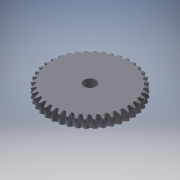
# Autodesk Inventor part: Worm Gear
Saved by Autodesk Inventor 2016 (Build 200138000, 138)
## iProperties
Created: 2015-06-13
Part Number: Worm Gear
Material: Steel, Mild
Document SubType Name: Modeling
Designer: steele
Categories: <?xml version="1.0" encoding="UTF-16"?> <MemberInstance><Categories><FamilyTemplate><FamilyTemplateParameter ValueType="xs:double" Id="1" ObjectReferenceKey="da_z" ObjectType="kUserParameterObject"/><FamilyTemplateParameter ValueType="xs:double" Id="2" ObjectReferenceKey="da_b" ObjectType="kUserParameterObject"/><FamilyTemplateParameter ValueType="xs:double" Id="3" ObjectReferenceKey="da_beta" ObjectType="kUserParameterObject"/><FamilyTemplateParameter ValueType="xs:double" Id="4" ObjectReferenceKey="da_m" ObjectType="kUserParameterObject"/><FamilyTemplateParameter ValueType="xs:double" Id="5" ObjectReferenceKey="da_alpha" ObjectType="kUserParameterObject"/><FamilyTemplateParameter ValueType="xs:double" Id="6" ObjectReferenceKey="da_da" ObjectType="kUserParameterObject"/><FamilyTemplateParameter ValueType="xs:double" Id="7" ObjectReferenceKey="da_aw" ObjectType="kUserParameterObject"/><FamilyTemplateParameter ValueType="xs:double" Id="8" ObjectReferenceKey="da_px" ObjectType="kUserParameterObject"/><FamilyTemplateParameter ValueType="xs:double" Id="9" ObjectReferenceKey="da_d" ObjectType="kUserParameterObject"/><FamilyTemplateParameter ValueType="xs:double" Id="10" ObjectReferenceKey="da_dae" ObjectType="kUserParameterObject"/><FamilyTemplateParameter ValueType="xs:double" Id="11" ObjectReferenceKey="da_fi" ObjectType="kUserParameterObject"/><FamilyTemplateParameter ValueType="xs:string" Id="12" ObjectReferenceKey="EAIAABAAAAAWFwAAAAAAAIAAAAAAAAAA" ObjectType="83910656" SubObjectId="SurfaceGeometry"/></FamilyTemplate><ParamToTemplateMap><ParamToTemplate CategoryParameter="//CategoryParameter[@InternalName='046C89C9-8512-4d59-83FE-43B91F4F132A']" TemplateParameter="1"/><ParamToTemplate CategoryParameter="//CategoryParameter[@InternalName='2552DF32-E462-4b46-AEBF-C6C7768E72AC']" TemplateParameter="2"/><ParamToTemplate CategoryParameter="//CategoryParameter[@InternalName='C9EE641D-15FC-4fae-A226-E94C4372FDD7']" TemplateParameter="3"/><ParamToTemplate><ParamToTemplate CategoryParameter="//CategoryParameter[@InternalName='00B6519A-459B-49c7-AD84-2E56D39A5744']" ConstantValue="0.000000"/></ParamToTemplate><ParamToTemplate><ParamToTemplate CategoryParameter="//CategoryParameter[@InternalName='04B31F0E-C7A6-4894-AA32-9629BEFACF47']" ConstantValue="1.000000"/></ParamToTemplate><ParamToTemplate><ParamToTemplate CategoryParameter="//CategoryParameter[@InternalName='43CBEC2E-7847-49e7-A936-2F7889FCB2D9']" ConstantValue="0.200000"/></ParamToTemplate><ParamToTemplate><ParamToTemplate CategoryParameter="//CategoryParameter[@InternalName='B1EFC894-105D-4ebd-86BF-FA20ED196853']" ConstantValue="0.266800"/></ParamToTemplate><ParamToTemplate><ParamToTemplate CategoryParameter="//CategoryParameter[@InternalName='51175063-3D10-4879-93E8-6246FE8B403D']" ConstantValue="2061532430.657340"/></ParamToTemplate><ParamToTemplate><ParamToTemplate CategoryParameter="//CategoryParameter[@InternalName='A3A52E27-4454-46a9-B0BD-C932399B70AF']" ConstantValue="0.300000"/></ParamToTemplate><ParamToTemplate CategoryParameter="//CategoryParameter[@InternalName='91B76062-C214-41d9-B1B9-14D2AB99603D']" TemplateParameter="4"/><ParamToTemplate CategoryParameter="//CategoryParameter[@InternalName='2D373A89-B862-43d6-8D0B-0CBF12AB9F6C']" TemplateParameter="5"/><ParamToTemplate CategoryParameter="//CategoryParameter[@InternalName='37777632-D6A2-4fac-9D53-DB8ACD95C989']" TemplateParameter="6"/><ParamToTemplate CategoryParameter="//CategoryParameter[@InternalName='FD1017F1-B727-4f7e-9707-0F86F1FF9423']" TemplateParameter="7"/><ParamToTemplate CategoryParameter="//CategoryParameter[@InternalName='3BF567DA-17EF-48d8-80EA-D119B07F6463']" TemplateParameter="8"/><ParamToTemplate CategoryParameter="//CategoryParameter[@InternalName='BF5A1E7E-5373-4a22-AAD3-F583781FCF3C']" TemplateParameter="9"/><ParamToTemplate CategoryParameter="//CategoryParameter[@InternalName='2A200944-5A8C-41ca-B96E-8520D2E510F1']" TemplateParameter="10"/><ParamToTemplate CategoryParameter="//CategoryParameter[@InternalName='E77AC4FD-7B43-4566-B0ED-7CA70B976BC8']" TemplateParameter="11"/><ParamToTemplate><ParamToTemplate CategoryParameter="//CategoryParameter[@InternalName='D4F72237-D604-435a-AD0B-F738B7463A00']" ConstantValue="110.000000"/></ParamToTemplate><ParamToTemplate><ParamToTemplate CategoryParameter="//CategoryParameter[@InternalName='9E1B4470-B2D3-4ff1-B813-535BB4CDF51A']" ConstantValue="1999479.615019"/></ParamToTemplate><ParamToTemplate><ParamToTemplate CategoryParameter="//CategoryParameter[@InternalName='A7A89E9A-52E6-4d4f-86CF-A81914F22AA4']" ConstantValue="250000000.000000"/></ParamToTemplate><ParamToTemplate><ParamToTemplate CategoryParameter="//CategoryParameter[@InternalName='B02FABAC-469F-4ad8-A219-DB4578299DF6']" ConstantValue="250000000.000000"/></ParamToTemplate><ParamToTemplate><ParamToTemplate CategoryParameter="//CategoryParameter[@InternalName='E6981962-40D5-4343-A0AD-C263FCC47E10']" ConstantValue="9.000000"/></ParamToTemplate><ParamToTemplate><ParamToTemplate CategoryParameter="//CategoryParameter[@InternalName='B958E99F-2BCD-4955-8634-793EB7B37B89']" ConstantValue="8.000000"/></ParamToTemplate><ParamToTemplate><ParamToTemplate CategoryParameter="//CategoryParameter[@InternalName='4AD49A87-569D-440f-A541-E3B52A6A9DCE']" ConstantValue="1219.200000"/></ParamToTemplate><ParamToTemplate><ParamToTemplate CategoryParameter="//CategoryParameter[@InternalName='4E5813A0-330D-4b41-BE23-D880B01A1D55']" ConstantValue="1654741.750360"/></ParamToTemplate><ParamToTemplate><ParamToTemplate CategoryParameter="//CategoryParameter[@InternalName='19EB8C86-AA88-4253-B4AA-2F5DF1CE171A']" ConstantValue="5515.805835"/></ParamToTemplate><ParamToTemplate CategoryParameter="//CategoryParameter[@InternalName='27C3BAF2-7550-4e4b-AE2C-0DB134B7D9B7']" TemplateParameter="12"/></ParamToTemplateMap><Category DisplayName="Gear" InternalName="DC85795E-93AB-48d5-8EEE-5A27447B64BD" Mnemonic="Gear"><CategoryParameter DisplayName="z" InternalName="046C89C9-8512-4d59-83FE-43B91F4F132A" Mnemonic="z"/><CategoryParameter DisplayName="b|.2|" InternalName="2552DF32-E462-4b46-AEBF-C6C7768E72AC" Mnemonic="b"/><CategoryParameter DisplayName="||b|" InternalName="C9EE641D-15FC-4fae-A226-E94C4372FDD7" Mnemonic="beta"/><CategoryParameter DisplayName="x" InternalName="00B6519A-459B-49c7-AD84-2E56D39A5744" Mnemonic="x"/><CategoryParameter DisplayName="a*" InternalName="04B31F0E-C7A6-4894-AA32-9629BEFACF47" Mnemonic="a"/><CategoryParameter DisplayName="c*" InternalName="43CBEC2E-7847-49e7-A936-2F7889FCB2D9" Mnemonic="c"/><CategoryParameter DisplayName="r|.f|*" InternalName="B1EFC894-105D-4ebd-86BF-FA20ED196853" Mnemonic="rf"/><CategoryParameter DisplayName="E" InternalName="51175063-3D10-4879-93E8-6246FE8B403D" Mnemonic="E"/><CategoryParameter DisplayName="||m|" InternalName="A3A52E27-4454-46a9-B0BD-C932399B70AF" Mnemonic="mi"/><Category DisplayName="WormGear" InternalName="1B25C7EF-093B-4025-B3D3-619CD2A4550C" Mnemonic="WormGear"><CategoryParameter DisplayName="m" InternalName="91B76062-C214-41d9-B1B9-14D2AB99603D" Mnemonic="m"/><CategoryParameter DisplayName="||a|" InternalName="2D373A89-B862-43d6-8D0B-0CBF12AB9F6C" Mnemonic="alpha"/><CategoryParameter DisplayName="d|.a|" InternalName="37777632-D6A2-4fac-9D53-DB8ACD95C989" Mnemonic="da"/><CategoryParameter DisplayName="a|.w|" InternalName="FD1017F1-B727-4f7e-9707-0F86F1FF9423" Mnemonic="aw"/><CategoryParameter DisplayName="p|.x|" InternalName="3BF567DA-17EF-48d8-80EA-D119B07F6463" Mnemonic="px"/><CategoryParameter DisplayName="d" InternalName="BF5A1E7E-5373-4a22-AAD3-F583781FCF3C" Mnemonic="d"/><CategoryParameter DisplayName="dae" InternalName="2A200944-5A8C-41ca-B96E-8520D2E510F1" Mnemonic="dae"/><CategoryParameter DisplayName="||d|" InternalName="E77AC4FD-7B43-4566-B0ED-7CA70B976BC8" Mnemonic="fi"/><CategoryParameter DisplayName="VHV" InternalName="D4F72237-D604-435a-AD0B-F738B7463A00" Mnemonic="VHV"/><CategoryParameter DisplayName="||s||.Hlim|" InternalName="9E1B4470-B2D3-4ff1-B813-535BB4CDF51A" Mnemonic="sHlim"/><CategoryParameter DisplayName="N|.Flim|" InternalName="A7A89E9A-52E6-4d4f-86CF-A81914F22AA4" Mnemonic="NFlim"/><CategoryParameter DisplayName="N|.Hlim|" InternalName="B02FABAC-469F-4ad8-A219-DB4578299DF6" Mnemonic="NHlim"/><CategoryParameter DisplayName="q|.F|" InternalName="E6981962-40D5-4343-A0AD-C263FCC47E10" Mnemonic="qF"/><CategoryParameter DisplayName="q|.H|" InternalName="B958E99F-2BCD-4955-8634-793EB7B37B89" Mnemonic="qH"/><CategoryParameter DisplayName="v|.max|" InternalName="4AD49A87-569D-440f-A541-E3B52A6A9DCE" Mnemonic="maxv"/><CategoryParameter DisplayName="S|.n|" InternalName="4E5813A0-330D-4b41-BE23-D880B01A1D55" Mnemonic="Sn"/><CategoryParameter DisplayName="K|.w|" InternalName="19EB8C86-AA88-4253-B4AA-2F5DF1CE171A" Mnemonic="Kw"/><CategoryParameter DisplayName="PitchDiameter" InternalName="27C3BAF2-7550-4e4b-AE2C-0DB134B7D9B7" Mnemonic="IDS_PITCHDIAM"/></Category></Category></Categories></MemberInstance>
Density: 7.86 g/cm^3
Appearance: Steel
CustomPartVersion: 1
Author: steele
Autodesk Inventor part; units mm, degrees
ref_plane "YZ Plane" through (0, 0, 0) normal (1, 0, 0) x (0, 1, 0)
ref_plane "XZ Plane" through (0, 0, 0) normal (0, 1, 0) x (-1, 0, 0)
ref_plane "XY Plane" through (0, 0, 0) normal (0, 0, 1) x (1, 0, 0)
ref_plane "Tooth Plane" through (0, -10, 0) normal (-0.0830455, 0, 0.9965458) x (0, 1, 0)
sketch "Base Body Sketch" plane through (0, 0, 0) normal (1, 0, 0) x (0, 1, 0)
  line L0 (0, -5.9267) -> (0, 5.9267) projected
  line L1 (0, 3.175) -> (20.8232, 3.175)
  line L2 (20.8232, 3.175) -> (22.7542, 2.2591)
  line L3 (-6.1383, 0) -> (36.83, 0) construction
  circle A0 centre (27.5167, 0) radius 5.2917
  line L4 (22.7542, 2.2591) -> (22.7542, -2.2591)
  line L5 (0, -3.175) -> (20.8232, -3.175)
  line L6 (0, 3.175) -> (0, -3.175)
  line L7 (20.8232, -3.175) -> (22.7542, -2.2591)
  dimension "d50" = 25.377
  dimension "d87" = 45.5083
  dimension "d89" = 10.5833
  dimension "d92" = 6.35
  dimension "d93" = 27.5167
  constraints: 14 end point, 3 symmetric about line, 2 perpendicular, 2 point on line, 1 centre point, 1 collinear
  measures "d50" angle of L2 L1
  measures "d87" diameter of L4 L0
  measures "d89" diameter of A0
  measures "d92" distance of L1.start L5.start
  measures "d93" distance from line of A0.centre L6
revolve "Base Body" add sketch "Base Body Sketch" angle 360 about axis through (0, 0, 0) along (0, 0, 1) picked at (22.6209, 0.3874) contours L0 L1 L2 A0 L7 L5 | A0 L2 L4 L7
revolve "Base Body2" cut sketch "Base Body Sketch" angle 360 about axis through (0, 0, 0) along (0, 0, 1) contours L7 L4 L2 A0 | A0 L2 L4 L7
sketch "Tooth Sketch" plane through (0, -10, 0) normal (-0.0830455, 0, 0.9965458) x (0, 1, 0)
  line L0 (10, 2.0436) -> (10, -2.0436) projected
  line L1 (-17.7707, 0) -> (-8.5843, 0) projected
  line L2 (-17.5167, 1.4597) -> (-17.5167, -1.4597)
  line L3 (-17.5167, -1.4597) -> (-12.4367, -1.4597)
  line L4 (-12.4367, -1.4597) -> (-9.8967, -0.5352)
  line L5 (-9.8967, -0.5352) -> (-9.8967, 0)
  line L6 (-9.8967, 0.5352) -> (-12.4367, 1.4597)
  line L7 (-12.4367, 1.4597) -> (-17.5167, 1.4597)
  line L8 (-9.8967, 0.5352) -> (-9.8967, 0)
  line L9 (-11.1667, 0) -> (-11.1667, -0.9975) construction
  dimension "d38" = 27.5167
  dimension "d39" = 20
  dimension "d40" = 5.08
  dimension "d41" = 6.35
  dimension "d42" = 0.9975
  constraints: 16 end point, 4 perpendicular, 3 equal length, 2 point on line, 1 midpoint, 1 parallel, 1 vertical
  measures "d38" distance between parallel lines of L0 L2
  measures "d39" angle of L6 L7
  measures "d40" distance of L6.end L2.start
  measures "d41" distance between parallel lines of L2 L9
  measures "d42" distance of L9.start L9.end
sketch "Sketch8" plane through (0, 0, 3.175) normal (0, 0, 1) x (1, 0, 0)
  circle A0 centre (0, 0) radius 20.8232 projected
  circle A1 centre (0, 0) radius 21.1667
  dimension "d77" = 42.3333
  constraints: 1 centre point, 1 coincident
  measures "d77" diameter of A1
surface extrude "Pitch Diameter" sketch "Sketch8" against normal blind 6.35 shown no curves A1
ref_plane "Work Plane13" through (0, 0, 0) normal (-0.0784591, 0.9969173, 0) x (0, 0, 1)
revolve "Tooth" cut sketch "Tooth Sketch" angle 360 about axis through (-1.4547, -27.5167, -0.1212) along (0.9965458, 0, 0.0830455)
pattern_circular "Tooth Pattern" count 40 over 360 about axis through (0, 0, 0) along (0, 0, 1) of "Tooth"
ref_plane "Work Plane14" through (0, 0, 0) normal (0.9969173, 0.0784591, 0) x (0, 0, 1)
ref_plane "Work Plane15" through (0, 0, 0) normal (0, -1, 0) x (0, 0, 1)
sketch "Sketch9" plane through (0, 0, 3.175) normal (0, 0, 1) x (0.9967613, -0.080417, 0)
  circle A0 centre (0, 0) radius 3.175
  dimension "d94" = 6.35
  constraints: 1 centre point, 1 coincident
  measures "d94" diameter of A0
extrude "Extrusion1" cut sketch "Sketch9" against normal through all
equation "\"d50\" = da_fi"
equation "\"d87\" = da_dae"
equation "\"d89\" = 2 * da_aw - da_da"
equation "\"d92\" = da_b"
equation "\"d93\" = da_aw"
equation "\"d38\" = da_aw"
equation "\"d39\" = da_alfat"
equation "\"d40\" = 0.5 * da_df1"
equation "\"d41\" = 0.5 * da_d1"
equation "\"d42\" = 0.3 * da_px"
equation "\"d77\" = da_dw"
equation "\"d78\" = da_b"
equation "\"da_aw\" = 27.51667"
equation "\"da_fi\" = 25.3769deg"
equation "\"da_b\" = 6.35"
equation "\"da_df\" = 39.79333"
equation "\"da_da\" = 44.45"
equation "\"da_beta\" = 4.763642deg"
equation "\"da_alfat\" = 20deg"
equation "\"da_df1\" = 10.16"
equation "\"da_da1\" = 14.81667"
equation "\"da_d1\" = 12.7"
equation "\"da_px\" = 3.32485"
equation "\"d68\" = da_aw"
equation "\"da_dw\" = 42.33333"
equation "\"da_rightdir\" = 0"
equation "\"d86\" = da_aw"
equation "\"da_dae\" = 45.50833"
body "Solid1"
body "Srf1"
